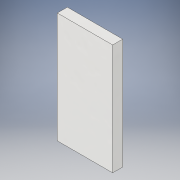
# Autodesk Inventor part: Perspex_window
Saved by Autodesk Inventor 2019 (Build 230136000, 136)
## iProperties
Created: 2020-02-17
Part Number: Perspex_window
Material: Generic
Document SubType Name: Modeling
Designer: craggles
Density: 1 g/cm^3
Appearance: Default
Author: craggles
Autodesk Inventor part; units mm, degrees
ref_plane "YZ Plane" through (0, 0, 0) normal (1, 0, 0) x (0, 1, 0)
ref_plane "XZ Plane" through (0, 0, 0) normal (0, 1, 0) x (-1, 0, 0)
ref_plane "XY Plane" through (0, 0, 0) normal (0, 0, 1) x (1, 0, 0)
sketch "Sketch1" plane through (0, 0, 0) normal (0, 1, 0) x (-1, 0, 0)
  line L0 (8.25, 1.5) -> (-8.25, 1.5)
  line L1 (-8.25, 1.5) -> (-8.25, -1.5)
  line L2 (-8.25, -1.5) -> (8.25, -1.5)
  line L3 (8.25, -1.5) -> (8.25, 1.5)
  point P0 (0, 0)
  point P1 (8.25, 0)
  point P2 (0, -1.5)
  dimension "d0" = 16.5
  dimension "d1" = 3
  constraints: 8 end point, 2 midpoint, 2 parallel, 1 horizontal, 1 horizontal alignment, 1 perpendicular, 1 vertical alignment
  measures "d0" distance of L2.end L1.end
  measures "d1" distance of L1.end L0.end
extrude "Extrusion1" add sketch "Sketch1" along normal blind 33
body "Solid1"
